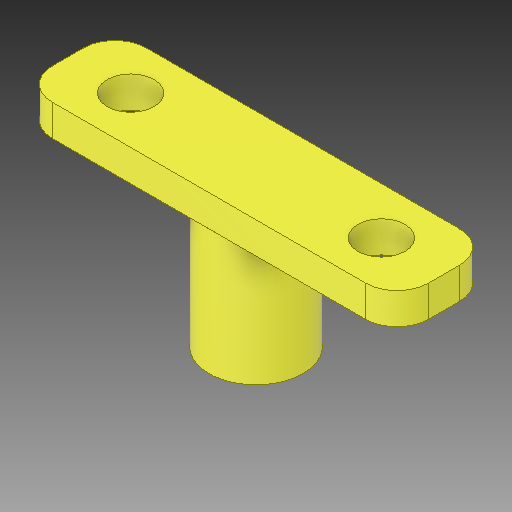
# Autodesk Inventor part: Shaft Encoder Adapter
Saved by Autodesk Inventor 2018.2 (Build 222227000, 227)
## iProperties
Created: 2018-02-08
Part Number: Shaft Encoder Adapter
Material: ABS Plastic
Document SubType Name: Modeling
Designer: Moochster
Density: 1.06 g/cm^3
Appearance: Smooth - Yellow
Mass: 0.45558 g
Surface Area: 6.24858 cm^2
Volume: 0.429793 cm^3
Author: Moochster
Autodesk Inventor part; units mm, degrees
ref_plane "YZ Plane" through (0, 0, 0) normal (1, 0, 0) x (0, 1, 0)
ref_plane "XZ Plane" through (0, 0, 0) normal (0, 1, 0) x (-1, 0, 0)
ref_plane "XY Plane" through (0, 0, 0) normal (0, 0, 1) x (1, 0, 0)
sketch "Sketch1" plane through (0, 0, 0) normal (0, 1, 0) x (-1, 0, 0)
  circle A0 centre (8, 0) radius 1.5
  circle A1 centre (-8, 0) radius 1.5
  line L0 (12, -3) -> (-12, -3)
  line L1 (-12, -3) -> (-12, 3)
  line L2 (-12, 3) -> (12, 3)
  line L3 (12, 3) -> (12, -3)
  circle A2 centre (0, 0) radius 1.4
  circle A3 centre (0, 0) radius 3
  point P0 (-12, 0)
  point P1 (0, 3)
  dimension "d0" = 3
  dimension "d1" = 3
  dimension "d2" = 8
  dimension "d3" = 8
  dimension "d4" = 24
  dimension "d5" = 6
  dimension "d6" = 2.8
  constraints: 8 end point, 4 centre point, 3 horizontal alignment, 2 coincident, 2 midpoint, 2 parallel, 1 horizontal, 1 perpendicular, 1 tangent, 1 vertical alignment
  measures "d0" diameter of A0
  measures "d1" diameter of A1
  measures "d2" distance of point (0, 0) A0.centre
  measures "d3" distance of A1.centre point (0, 0)
  measures "d4" distance of L1.end L2.end
  measures "d5" distance of L0.end L1.end
  measures "d6" diameter of A2
extrude "Extrusion1" add sketch "Sketch1" along normal blind 2 contours L0 A3 L2 L3 | L0 L1 L2 A3 | A3 | A2
extrude "Extrusion2" add sketch "Sketch1" against normal blind 8 contours A3
fillet "Fillet2" radius 2 4 edges at (-12, 1, 3) (-12, 1, -3) (12, 1, 3) (12, 1, -3)
body "Solid1"
